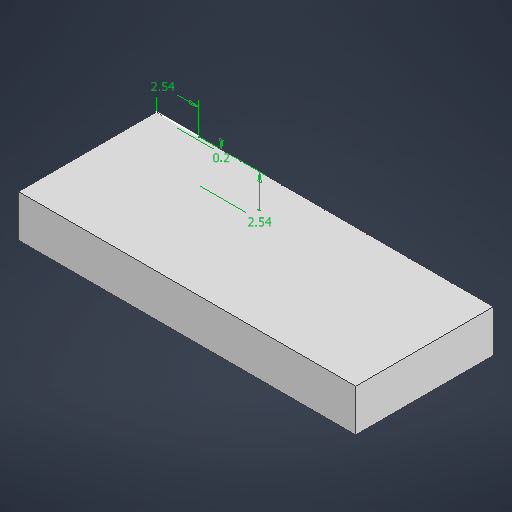
# Autodesk Inventor part: CasePinos
Saved by Autodesk Inventor 2026.2 (Build 302298010, 298A)
## iProperties
Created: 2026-04-17
Part Number: CasePinos
Material: Generic
Document SubType Name: Modeling
Designer: mrcm
Density: 1 g/cm^3
Appearance: Default
Author: mrcm
Autodesk Inventor part; units mm, degrees
ref_plane "YZ Plane" through (0, 0, 0) normal (1, 0, 0) x (0, 1, 0)
ref_plane "XZ Plane" through (0, 0, 0) normal (0, 1, 0) x (-1, 0, 0)
ref_plane "XY Plane" through (0, 0, 0) normal (0, 0, 1) x (1, 0, 0)
sketch "Sketch1" plane through (0, 0, 0) normal (0, 0, 1) x (1, 0, 0)
  line L0 (-1.27, -1.27) -> (1.27, -1.27)
  line L1 (1.27, -1.27) -> (1.27, 1.27)
  line L2 (1.27, 1.27) -> (-1.27, 1.27)
  line L3 (-1.27, 1.27) -> (-1.27, -1.27)
  line L4 (-1.27, -1.27) -> (1.27, 1.27) construction
  line L5 (1.27, -1.27) -> (-1.27, 1.27) construction
  line L6 (-1.07, 1.07) -> (1.07, 1.07)
  line L7 (1.07, 1.07) -> (1.07, -1.07)
  line L8 (1.07, -1.07) -> (-1.07, -1.07)
  line L9 (-1.07, -1.07) -> (-1.07, 1.07)
  point P0 (0, 0)
  point P1 (0, 1.07)
  dimension "d0" = 2.54
  dimension "d1" = 2.54
  dimension "d2" = 0.2
  constraints: 20 end point, 4 parallel, 3 midpoint, 2 perpendicular, 1 horizontal, 3 other
  measures "d0" distance between parallel lines of L0 L2
  measures "d1" distance between parallel lines of L3 L1
  measures "d2" distance from line of point (0, 1.07) L2
extrude "Extrusion1" add sketch "Sketch1" along normal blind 8.3 contours L3 L2 L1 L0 | L6 L7 L8 L9
shell "Shell1" thickness 0.4 removed faces 1 at (0.4233, -0.4233, 0)
chamfer "Chamfer1" distance 0.4 angle 45 4 edges at (0, -0.87, 0) (-0.87, 0, 0) (0, 0.87, 0) (0.87, 0, 0)
pattern_linear "Rectangular Pattern1" count 8 spacing 2.54 along (1, 0, 0)
body "Solid1"
